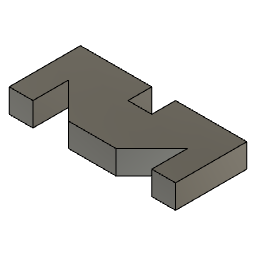
Model 11 (Autodesk Fusion 360 design; units mm, degrees)
Autodesk Fusion 360 part; units mm, degrees
sketch "Sketch1" plane through (0, 0, 0) normal (0, 0, 1) x (1, 0, 0)
  line L0 (0, 0) -> (0, 30)
  line L1 (0, 30) -> (30, 30)
  line L2 (30, 30) -> (30, 20)
  line L3 (30, 20) -> (35, 20)
  line L4 (35, 20) -> (35, 0)
  line L5 (0, 0) -> (10, 0)
  line L6 (10, 0) -> (10, 15)
  line L7 (35, 0) -> (25, 0)
  line L8 (25, 0) -> (10, 15)
  dimension "d1" = 30
  dimension "d2" = 30
  dimension "d3" = 10
  dimension "d4" = 5
  dimension "d5" = 20
  dimension "d6" = 15
  dimension "d7" = 10
  dimension "d8" = 15
  constraint coincident L0.start L5.start
  constraint vertical L0
  constraint perpendicular L0 L1
  constraint perpendicular L1 L2
  constraint perpendicular L2 L3
  constraint perpendicular L3 L4
  constraint perpendicular L0 L5
  constraint perpendicular L5 L6
  constraint perpendicular L4 L7
  measures "d1" distance of L0.start L0.end
  measures "d2" distance of L0.end L1.end
  measures "d3" distance of L1.end L2.end
  measures "d4" distance of L2.end L3.end
  measures "d5" distance of L3.end L4.end
  measures "d6" distance of L5.end L6.end
  measures "d7" distance of L4.end L7.end
  measures "d8" distance of L6 L7.end
extrude "Extrude1" add sketch "Sketch1" along normal blind 10
mirror "Mirror1" about plane through (35, 20, 0) normal (1, 0, 0) of bodies 1 merged
